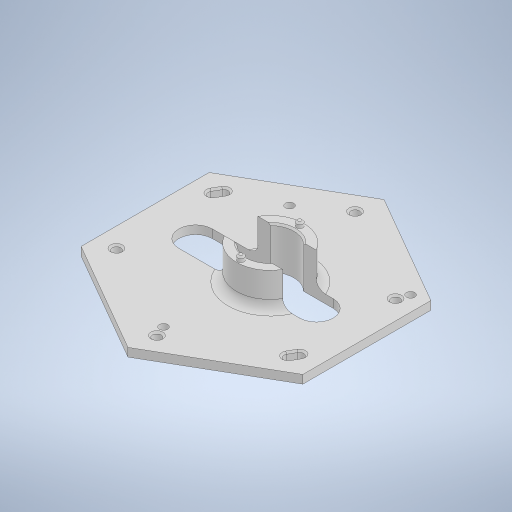
# Autodesk Inventor part: pi_case_top
Saved by Autodesk Inventor 2024 (Build 280153000, 153)
## iProperties
Created: 2024-03-18
Part Number: pi_case_top
Material: 일반
Document SubType Name: Modeling
Designer: SSAFY
Density: 1 g/cm^3
Appearance: 기본값
Author: SSAFY
Autodesk Inventor part; units mm, degrees
ref_plane "YZ Plane" through (0, 0, 0) normal (1, 0, 0) x (0, 1, 0)
ref_plane "XZ Plane" through (0, 0, 0) normal (0, 1, 0) x (-1, 0, 0)
ref_plane "XY Plane" through (0, 0, 0) normal (0, 0, 1) x (1, 0, 0)
sketch "스케치2" plane through (0, 0, 0) normal (0, 1, 0) x (-1, 0, 0)
  line L0 (0, 70.4) -> (60.9682, 35.2)
  line L1 (60.9682, 35.2) -> (60.9682, -35.2)
  line L2 (60.9682, -35.2) -> (0, -70.4)
  line L3 (0, -70.4) -> (-60.9682, -35.2)
  line L4 (-60.9682, -35.2) -> (-60.9682, 35.2)
  line L5 (-60.9682, 35.2) -> (0, 70.4)
  line L6 (0, 76.1735) -> (65.9682, 38.0868)
  line L7 (65.9682, 38.0868) -> (65.9682, -38.0868)
  line L8 (65.9682, -38.0868) -> (0, -76.1735)
  line L9 (0, -76.1735) -> (-65.9682, -38.0868)
  line L10 (-65.9682, -38.0868) -> (-65.9682, 38.0868)
  line L11 (-65.9682, 38.0868) -> (0, 76.1735)
  point P0 (0, 0)
  point P1 (0, 0)
  dimension "d0" = 5
  dimension "d1" = 70.4
  constraints: 24 end point, 1 coincident, 18 other
  measures "d0" distance between parallel lines of L10 L4
  measures "d1" distance of L0.end L1.end
extrude "돌출1" add sketch "스케치2" along normal blind 5 contours L0 L1 L2 L3 L4 L5 | L6 L7 L8 L9 L10 L11
sketch "스케치3" plane through (0, 5, 0) normal (0, 1, 0) x (1, 0, 0)
  circle A0 centre (8.5, 0) radius 14.06
  circle A1 centre (8.5, 0) radius 20.06
  line L0 (-8.8898, 10) -> (25.8898, 10)
  line L1 (-8.8898, -10) -> (25.8898, -10)
  point P0 (0, 0)
  point P1 (-1.3835, -10)
  point P2 (18.3835, -10)
  point P3 (-1.3835, 10)
  point P4 (18.3835, 10)
  dimension "d4" = 28.12
  dimension "d5" = 6
  dimension "d6" = 10
  dimension "d7" = 10
  dimension "d8" = 8.5
  constraints: 4 end point, 4 point on circle, 2 centre point, 2 horizontal
  measures "d4" diameter of A0
  measures "d5" radial gap between concentric circles of A0 A1
  measures "d6" distance from line of L0 A0.centre
  measures "d7" distance from line of L1 A0.centre
  measures "d8" distance of A0.centre point (0, 0)
extrude "돌출2" add sketch "스케치3" along normal blind 20 contours A0 L0 A1 | L1 A1 A0
sketch "스케치4" plane through (0, 25, 0) normal (0, 1, 0) x (1, 0, 0)
  arc A0 (18.3835, 10) -> (-1.3835, 10) centre (8.5, 0) ccw construction
  arc A1 (25.8898, 10) -> (-8.8898, 10) centre (8.5, 0) ccw construction
  circle A2 centre (8.5, -17.5) radius 2
  line L0 (0, 0) -> (8.5, 0) construction
  circle A3 centre (8.5, 17.5) radius 2
  dimension "d11" = 17.5
  dimension "d12" = 4
  constraints: 2 centre point, 2 end point, 1 horizontal, 1 symmetric about line, 1 other
  measures "d11" distance of A0.centre A2.centre
  measures "d12" diameter of A2
extrude "돌출3" add sketch "스케치4" along normal blind 3
sketch "스케치5" plane through (0, 5, 0) normal (0, 1, 0) x (1, 0, 0)
  arc A0 (-1.3835, -10) -> (18.3835, -10) centre (8.5, 0) ccw construction
  circle A1 centre (0, -55) radius 2.5
  circle A2 centre (-25, 45) radius 2.5
  circle A3 centre (57, 35) radius 2.5
  point P0 (0, 0)
  dimension "d15" = 5
  dimension "d16" = 55
  dimension "d17" = 5
  dimension "d18" = 45
  dimension "d19" = 25
  dimension "d20" = 5
  dimension "d21" = 57
  dimension "d22" = 35
  constraints: 3 centre point
  measures "d15" diameter of A1
  measures "d16" distance of A1.centre point (0, 0)
  measures "d17" diameter of A2
  measures "d18" vertical distance of A2.centre point (0, 0)
  measures "d19" horizontal distance of point (0, 0) A2.centre
  measures "d20" diameter of A3
  measures "d21" horizontal distance of A3.centre point (0, 0)
  measures "d22" vertical distance of A3.centre A0.centre
extrude "돌출4" cut sketch "스케치5" against normal through all
sketch "스케치6" plane through (0, 5, 0) normal (0, 1, 0) x (1, 0, 0)
  arc A0 (18.3835, 10) -> (-1.3835, 10) centre (8.5, 0) ccw construction
  circle A1 centre (8.5, 0) radius 14.06
  line L0 (65.9682, -38.0868) -> (65.9682, 38.0868) construction
  line L1 (-65.9682, 38.0868) -> (-65.9682, -38.0868) construction
  line L2 (-1.3835, 10) -> (-45.9682, 10)
  line L3 (-1.3835, -10) -> (-45.9682, -10)
  line L4 (-45.9682, -10) -> (-45.9682, 10)
  line L5 (18.3835, 10) -> (45.9682, 10)
  line L6 (45.9682, 10) -> (45.9682, -10)
  line L7 (45.9682, -10) -> (18.3835, -10)
  point P0 (0, 0)
  dimension "d27" = 20
  dimension "d28" = 20
  constraints: 12 end point, 3 horizontal, 3 perpendicular, 2 point on circle, 1 centre point, 1 coincident, 1 point on line
  measures "d27" distance between parallel lines of L0 L6
  measures "d28" distance between parallel lines of L4 L1
extrude "돌출5" cut sketch "스케치6" against normal through all
sketch "스케치7" plane through (0, 5, 0) normal (0, 1, 0) x (1, 0, 0)
  line L0 (0, 60) -> (51.9615, 30)
  line L1 (51.9615, 30) -> (51.9615, -30)
  line L2 (51.9615, -30) -> (0, -60)
  line L3 (0, -60) -> (-51.9615, -30)
  line L4 (-51.9615, -30) -> (-51.9615, 30)
  line L5 (-51.9615, 30) -> (0, 60)
  line L6 (-56.9615, 32.8868) -> (-56.9615, -32.8868)
  line L7 (-56.9615, -32.8868) -> (0, -65.7735)
  line L8 (0, -65.7735) -> (56.9615, -32.8868)
  line L9 (56.9615, -32.8868) -> (56.9615, 32.8868)
  line L10 (56.9615, 32.8868) -> (0, 65.7735)
  line L11 (0, 65.7735) -> (-56.9615, 32.8868)
  line L12 (-56.9615, 32.8868) -> (56.9615, -32.8868)
  line L13 (0, 65.7735) -> (0, -65.7735)
  line L14 (-56.9615, -32.8868) -> (56.9615, 32.8868)
  circle A0 centre (-54.4615, 28.5566) radius 2.5
  circle A1 centre (-51.9615, 32.8868) radius 2.5
  circle A2 centre (-54.4615, -28.5566) radius 2.5
  circle A3 centre (-2.5, 61.4434) radius 2.5
  circle A4 centre (-51.9615, 32.8868) radius 2.6
  circle A5 centre (-54.4615, 28.5566) radius 2.6
  circle A6 centre (-54.4615, -28.5566) radius 2.6
  circle A7 centre (-2.5, 61.4434) radius 2.6
  line L15 (-28.4808, -49.3301) -> (28.4808, 49.3301)
  circle A8 centre (54.4615, -28.5566) radius 2.6
  circle A9 centre (51.9615, -32.8868) radius 2.6
  circle A10 centre (2.5, -61.4434) radius 2.6
  circle A11 centre (54.4615, 28.5566) radius 2.6
  line L16 (-54.2132, 34.1868) -> (-56.9615, 29.4265)
  line L17 (-52.2099, 27.2566) -> (-49.7099, 31.5868)
  line L18 (56.7132, -29.8566) -> (53.9649, -34.6169)
  line L19 (49.7099, -31.5868) -> (52.2099, -27.2566)
  point P0 (0, 0)
  point P1 (0, 0)
  point P2 (51.9615, 27.8425)
  point P3 (56.9615, 27.8425)
  point P4 (56.9615, 29.2708)
  point P5 (53.83, 31.0788)
  point P6 (52.5931, 30.3646)
  point P7 (51.9615, 29.2708)
  point P8 (51.9615, -29.2708)
  point P9 (52.5931, -30.3646)
  point P10 (53.83, -31.0788)
  point P11 (56.9615, -29.2708)
  point P12 (56.9615, -27.8425)
  point P13 (51.9615, -27.8425)
  point P14 (0.6315, -59.6354)
  point P15 (0, -60.7292)
  point P16 (0, -62.1575)
  point P17 (3.1315, -63.9655)
  point P18 (4.3685, -63.2514)
  point P19 (1.8685, -58.9212)
  point P20 (-53.83, 31.0788)
  point P21 (-52.5931, 30.3646)
  point P22 (54.2132, -34.1868)
  point P23 (-56.7132, 29.8566)
  dimension "d29" = 60
  dimension "d30" = 5
  dimension "d31" = 5
  dimension "d32" = 5
  dimension "d33" = 5
  dimension "d34" = 5
  dimension "d35" = 5.2
  dimension "d36" = 0.1
  dimension "d37" = 5.2
  dimension "d38" = 5.2
  constraints: 40 end point, 11 centre point, 10 tangent, 8 symmetric about line, 2 coincident, 2 midpoint, 2 point on circle, 1 parallel, 1 point on line, 27 other
  measures "d29" distance of L3.end L4.end
  measures "d30" distance between parallel lines of L4 L6
  measures "d31" diameter of A0
  measures "d32" diameter of A1
  measures "d33" diameter of A2
  measures "d34" diameter of A3
  measures "d35" diameter of A4
  measures "d37" diameter of A6
  measures "d38" diameter of A7
extrude "돌출6" cut sketch "스케치7" against normal through all contours A7 L5 | L5 A3 L13 A7 | L13 A7 | L5 A7 L11 A3 | A3 | A3 L11 A7 L13 | L17 L4 A5 L12 | L12 L5 A4 L17 | L19 L1 A8 L12 | L12 L2 A9 L19 | A11 L14 L9 L1 | L1 A11 | A11 L14 | L11 A7 | L5 A4 L17 | L12 A4 L5 | L4 A5 L12 | L17 A5 L4 | L12 A9 L2 | L1 A8 L12 | L2 A9 L19 | L19 A8 L1 | A10 L2 | L2 A10 L8 L13 | L13 A10 | A6 L14 A2 L4 | L4 A6 | A6 L14 | A11 L9 | A4 L5 | L5 A1 L11 A4 | L11 A4 | A5 L4 | L4 A0 A4 A5 | A4 A5 A1 L5 | A4 A0 L12 | L12 A1 A5 | L4 A2 L6 A6 | A5 L6 A0 L4 | A8 L1 | L1 A8 L9 A9 | A9 A8 L8 L2 | L2 A9 | A9 L12 | L12 A8 | A2 | L14 A6 L6 A2 | A1 A5 | A1 A5 A4 L11 | A0 A4 | A0 A4 L12 | A0 A4 | L12 A5 A1 | A1 A5 | L6 A6 | A5 L6 | A8 L18 L12 | L12 L18 A9 | L8 A9 | A8 L9 | L8 A10 | A4 L12 L16 | L6 A5 A4 A0 | A5 L16 L12
fillet "모깎기1" radius 5 2 edges at (8.5, 5, 20.06) (8.5, 5, -20.06)
chamfer "모따기1" distance 1 angle 45 19 edges at (8.5, 25, 14.06) (8.5, 25, -14.06) (6.5, 28, -17.5) (6.5, 28, 17.5) (55.7615, 5, 26.305) (55.4632, 5, 32.0217) (50.6615, 5, 35.1384) (50.9599, 5, 29.4217) (-50.6615, 5, -35.1384) (-50.9599, 5, -29.4217) (-55.7615, 5, -26.305) (-55.4632, 5, -32.0217) (-57.0615, 5, 28.5566) (-5.1, 5, -61.4434) (0.6315, 5, 59.6354) (-27.5, 0, -45) (55.0931, 5, -26.0345) (-2.5, 0, 55) (54.5, 0, -35)
fillet "모깎기2" radius 10 4 edges at (-45.9682, 2.5, -10) (-45.9682, 2.5, 10) (45.9682, 2.5, -10) (45.9682, 2.5, 10)
